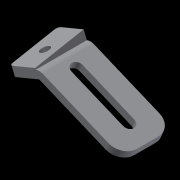
# Autodesk Inventor part: HipBottomConnectorLeftNew
Saved by Autodesk Inventor 2015 SP1 (Build 190203100, 203)
## iProperties
Created: 2014-08-29
Part Number: HipBottomConnectorLeftNew
Material: Generic
Document SubType Name: Modeling
Designer: Inventor
Mass: 4.04758 g
Surface Area: 38.1663 cm^2
Volume: 4.04758 cm^3
Density: 1 g/cm^3
Appearance: Default
Author: Inventor
Autodesk Inventor part; units mm, degrees
ref_plane "YZ Plane" through (0, 0, 0) normal (1, 0, 0) x (0, 1, 0)
ref_plane "XZ Plane" through (0, 0, 0) normal (0, 1, 0) x (-1, 0, 0)
sketch "Base" plane through (0, 0, 0) normal (0, 0, 1) x (1, 0, 0)
  line L0 (14, -3) -> (44, -3)
  line L1 (14, 3) -> (44, 3)
  arc A0 (44, -3) -> (44, 3) centre (44, 0) ccw
  arc A1 (14, 3) -> (14, -3) centre (14, 0) ccw
  line L2 (55, 13.75) -> (-10, 13.75)
  line L3 (55, -13.75) -> (55, 13.75)
  line L4 (-10, -13.75) -> (55, -13.75)
  line L5 (44, 0) -> (0, 0) construction
  line L6 (-10, 13.75) -> (-10, -13.75)
  dimension "d1" = 27.5
  dimension "d4" = 30
  dimension "d5" = 13.75
  dimension "d6" = 65
  dimension "d7" = 11
  dimension "d15" = 3
  constraints: 14 end point, 4 point on circle, 3 horizontal, 3 tangent, 2 centre point, 2 parallel, 2 vertical, 1 coincident, 1 equal radius, 1 other
  measures "d1" distance between parallel lines of L4 L2
  measures "d4" distance of L1.start L1.end
  measures "d5" distance between parallel lines of L4 L5
  measures "d6" distance of L2.start L2.end
  measures "d7" distance from line of L1.end L3
  measures "d15" radius of A0
extrude "BaseFeature" add sketch "Base" along normal mid plane 4
fillet "BaseFilletFeature" radius 8 2 edges at (55, -13.75, 0) (55, 13.75, 0)
fillet "BaseFillet2Feature" radius 2 2 edges at (-10, 13.75, 0) (-10, -13.75, 0)
sketch "BaseBend" plane through (0, 0, 2) normal (0, 0, 1) x (1, 0, 0)
  line L0 (-10, 11.75) -> (-10, -11.75) construction
  line L1 (7, 13.75) -> (7, -13.75)
  line L2 (-8, -13.75) -> (47, -13.75) construction
  line L3 (47, 13.75) -> (-8, 13.75) construction
  dimension "d12" = 17
  constraints: 2 end point, 2 point on line, 1 vertical
  measures "d12" distance between parallel lines of L1 L0
bend part "BaseBendFeature" radius 5 angle 45 line through (7, 13.75, 2) along (0, -1, 0) centre toward (0, 0, -1) moving side (1, 0, 0) both sides yes
ref_plane "ConnectorPlatePlane" through (-21.865, 84.6972, 5.9274) normal (0.3790943, 0.1366374, -0.9152146) x (0.9238795, 0, 0.3826834)
sketch "ConnectorPlateSpacer" plane through (5.0866, -13.75, 1.6194) normal (-0.3826834, 0, 0.9238795) x (0.9238795, 0, 0.3826834)
  line L0 (0, 0) -> (0, 27.5) projected
  line L1 (0, 27.5) -> (-13.0365, 27.5) projected
  arc A0 (-13.0365, 27.5) -> (-15.0365, 25.5) centre (-13.0365, 25.5) ccw projected
  line L2 (-15.0365, 25.5) -> (-15.0365, 2) projected
  arc A1 (-15.0365, 2) -> (-13.0365, 0) centre (-13.0365, 2) ccw projected
  line L3 (-13.0365, 0) -> (0, 0) projected
  point P0 (-5.3191, 13.75)
extrude "ConnectorPlateSpacerFeature" add sketch "ConnectorPlateSpacer" along normal up to surface surface through (-21.865, 84.6972, 5.9274) normal (0.3790943, 0.1366374, -0.9152146)
sketch "Sketch4" plane through (4.8129, -13.75, 2.28) normal (-0.3790943, -0.1366374, 0.9152146) x (0.9238795, 0, 0.3826834)
  circle A0 centre (-6.9707, 12.4795) radius 3 projected
hole "ConnectorPlateHole" at (-2.2797, -1.3875, 1.1878) direction (0.3790943, 0.1366374, -0.9152146) diameter 5 end through all
equation "\"d5\" = 0.5 * d1"
body "Solid1"
